Back Brace (Autodesk Fusion 360 design; units mm, degrees)
Autodesk Fusion 360 part; units mm, degrees
sketch "Sketch1" plane through (0, 0, 0) normal (0, 0, 1) x (1, 0, 0)
  line L0 (0, 0) -> (-148, 0)
  line L1 (-148, 0) -> (-148, 57)
  line L2 (-78, 127) -> (-70, 127)
  line L3 (0, 57) -> (0, 0)
  arc A0 (0, 57) -> (-70, 127) centre (-70, 57) ccw
  arc A1 (-78, 127) -> (-148, 57) centre (-78, 57) ccw
  point P0 (0, 127)
  dimension "d1" = 148
  dimension "d2" = 127
  dimension "d3" = 70
  constraint horizontal L0
  constraint vertical L1
  constraint horizontal L2
  constraint vertical L3
  constraint coincident L0.start L3.end
  constraint coincident P0 L2
  constraint coincident P0 L3
  constraint tangent L2 A0
  constraint tangent L3 A0
  constraint tangent L1 A1
  constraint tangent L2 A1
  constraint equal A0 A1
  measures "d1" distance of L0.start L0.end
  measures "d2" distance of L0.start P0
  measures "d3" radius of A0
extrude "Extrude1" add sketch "Sketch1" along normal blind 2
